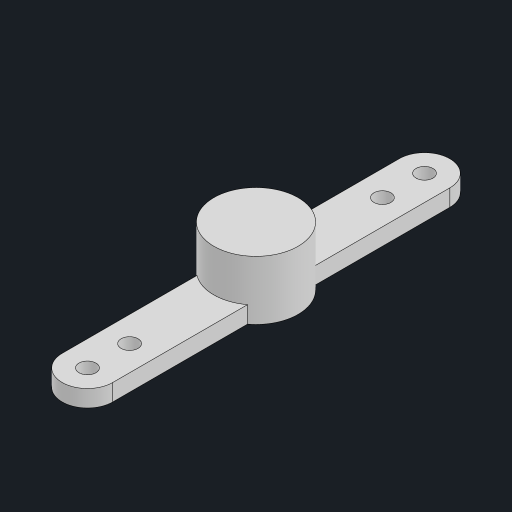
# Autodesk Inventor part: ナックル
Saved by Autodesk Inventor 2023 (Build 270158000, 158)
## iProperties
Created: 2022-06-07
Part Number: ナックル
Material: Generic
Document SubType Name: Modeling
Designer: legot
Density: 1 g/cm^3
Appearance: Default
Author: legot
Autodesk Inventor part; units mm, degrees
ref_plane "YZ Plane" through (0, 0, 0) normal (1, 0, 0) x (0, 1, 0)
ref_plane "XZ Plane" through (0, 0, 0) normal (0, 1, 0) x (-1, 0, 0)
ref_plane "XY Plane" through (0, 0, 0) normal (0, 0, 1) x (1, 0, 0)
sketch "スケッチ1" plane through (0, 0, 0) normal (0, 1, 0) x (-1, 0, 0)
  circle A0 centre (0, 0) radius 2.5
  circle A1 centre (0, 10) radius 1.5
  circle A2 centre (0, -10) radius 1.5
  line L0 (1.5, 10) -> (1.5, 2)
  line L1 (-1.5, 10) -> (-1.5, 2)
  line L2 (-1.5, -2) -> (-1.5, -10)
  line L3 (1.5, -2) -> (1.5, -10)
  dimension "d0" = 5
  dimension "d1" = 3
  dimension "d2" = 3
  dimension "d3" = 10
  dimension "d4" = 10
  constraints: 8 end point, 8 point on circle, 4 tangent, 4 vertical, 3 centre point, 2 vertical alignment, 1 coincident
  measures "d0" diameter of A0
  measures "d1" diameter of A1
  measures "d2" diameter of A2
  measures "d3" distance of point (0, 0) A1.centre
  measures "d4" distance of A2.centre point (0, 0)
extrude "押し出し1" add sketch "スケッチ1" along normal blind 1
sketch "スケッチ2" plane through (0, 1, 0) normal (0, 1, 0) x (1, 0, 0)
  arc A0 (-1.5, 2) -> (-1.5, -2) centre (0, 0) ccw projected
  circle A1 centre (0, 0) radius 2.5 projected
extrude "押し出し2" add sketch "スケッチ2" along normal blind 2.5
sketch "スケッチ3" plane through (0, 0, 0) normal (0, -1, 0) x (1, 0, 0)
  arc A0 (1.5, 10) -> (-1.5, 10) centre (0, 10) ccw projected
  arc A1 (-1.5, -10) -> (1.5, -10) centre (0, -10) ccw projected
  point P0 (0, 7.5)
  point P1 (0, -7.5)
  dimension "d9" = 2.5
  dimension "d10" = 2.5
  constraints: 2 coincident, 2 vertical alignment
  measures "d9" distance of point (0, 7.5) point (0, 10)
  measures "d10" distance of point (0, -7.5) point (0, -10)
hole "穴1" at (0, 0, 10) at (0, 0, -10) at (0, 0, 7.5) at (0, 0, -7.5) direction (0, 1, 0) diameter 1 end through all
equation "\"d4\" = d3"
equation "\"d10\" = d9"
